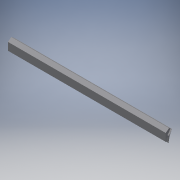
# Autodesk Inventor part: junta auto falante
Saved by Autodesk Inventor 2016 (Build 200138000, 138)
## iProperties
Created: 2017-06-08
Part Number: junta auto falante
Material: Genérico
Document SubType Name: Modeling
Designer: Fabio
Density: 1 g/cm^3
Appearance: Padrão
Author: Fabio
Autodesk Inventor part; units mm, degrees
ref_plane "YZ Plane" through (0, 0, 0) normal (1, 0, 0) x (0, 1, 0)
ref_plane "XZ Plane" through (0, 0, 0) normal (0, 1, 0) x (-1, 0, 0)
ref_plane "XY Plane" through (0, 0, 0) normal (0, 0, 1) x (1, 0, 0)
sketch "Esboço1" plane through (0, 0, 0) normal (1, 0, 0) x (0, 1, 0)
  line L0 (-10.3551, -6.5909) -> (-10.3551, 9.4091)
  line L1 (-10.3551, -6.5909) -> (-8.3551, -6.5863)
  line L2 (-8.3551, -6.5863) -> (-8.3551, -0.5863)
  line L3 (-8.3551, -0.5863) -> (-4.3551, -0.5863)
  line L4 (-4.3551, -0.5863) -> (-4.3551, -11.8863)
  line L5 (-4.3551, -11.8863) -> (-4.3551, -11.8863)
  line L6 (-3.45, 14.9711) -> (-10.3551, 9.4091)
  line L7 (-0.4417, 12.7091) -> (-7.0405, 3.4271)
  line L8 (-7.0405, 3.4271) -> (-3.7804, 1.1094)
  line L9 (-3.45, 14.9711) -> (-0.4417, 12.7091)
  line L10 (-3.7804, 1.1094) -> (2.7554, 10.3053)
  arc A0 (2.7554, 10.3053) -> (-4.3551, -11.8863) centre (37.3986, -13.0299) ccw
  dimension "d8" = 16
  dimension "d13" = 2
  dimension "d14" = 6
  dimension "d15" = 4
  dimension "d16" = 0
  dimension "d17" = 4
  dimension "d18" = 11.3
  dimension "d19" = 6
  dimension "d25" = 4
  dimension "d27" = 4
  constraints: 22 end point, 2 point on circle, 2 vertical, 1 centre point, 1 perpendicular
  measures "d8" distance of L0.start L0.end
  measures "d13" distance of L0.start L1.end
  measures "d14" distance of L1.end L2.end
  measures "d15" distance of L3.end L2.end
  measures "d16" distance of L4.end L5.end
  measures "d17" distance of L3.end L2.end
  measures "d18" distance of L3.end L4.end
  measures "d19" distance of L1.end L2.end
  measures "d25" distance of L7.end L8.end
  measures "d27" distance of L10.end L7.start
extrude "Extrusão1" add sketch "Esboço1" along normal blind 330
